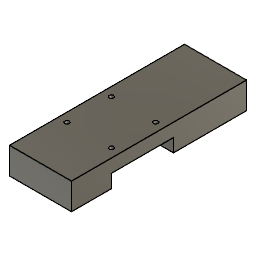
assembly (Autodesk Fusion 360 archive; units mm, degrees)
design "2x4_v2"
part number: 2026-04-10-14-49-08-842
Autodesk Fusion 360 part; units mm, degrees
sketch "Sketch1" plane through (0, 0, 0) normal (0, 0, 1) x (1, 0, 0)
  line L0 (0, 0) -> (88.9, 0)
  line L1 (88.9, 0) -> (88.9, 250.825)
  line L2 (88.9, 250.825) -> (0, 250.825)
  line L3 (0, 250.825) -> (0, 0)
  line L4 (0, 57.15) -> (88.9, 57.15)
  line L5 (0, 146.05) -> (88.9, 146.05)
  dimension "d1" = 88.9
  dimension "d2" = 250.825
  dimension "d3" = 57.15
  dimension "d4" = 88.9
  constraint horizontal L0
  constraint vertical L1
  constraint horizontal L2
  constraint vertical L3
  constraint coincident L0.start L3.end
  constraint coincident L3 L4.start
  constraint coincident L1 L4.end
  constraint perpendicular L1 L4
  constraint coincident L3 L5.start
  constraint coincident L1 L5.end
  constraint perpendicular L1 L5
  measures "d1" distance of L0.start L0.end
  measures "d2" distance of L0.end L1.end
  measures "d3" distance of L0 L4
  measures "d4" distance of L4 L5
extrude "Extrude1" add sketch "Sketch1" along normal blind 38.1
extrude "Extrude2" cut sketch "Sketch1" along normal blind 19.05 contours L1 L3 L4 L5
sketch "Sketch2" plane through (0, 0, 19.05) normal (0, 0, -1) x (1, 0, 0)
  line L0 (88.9, -57.15) -> (0, -57.15)
  line L1 (0, -57.15) -> (0, -146.05)
  line L2 (0, -146.05) -> (88.9, -146.05)
  line L3 (88.9, -146.05) -> (88.9, -57.15)
  line L4 (12.7, -133.35) -> (76.2, -133.35)
  line L5 (76.2, -133.35) -> (76.2, -69.85)
  line L6 (76.2, -69.85) -> (12.7, -69.85)
  line L7 (12.7, -69.85) -> (12.7, -133.35)
  dimension "d9" = -12.7
hole "Hole1" at (76.2, 69.85, 19.05) at (76.2, 133.35, 19.05) at (12.7, 133.35, 19.05) at (12.7, 69.85, 19.05) direction (0, 0, 1) diameter 6.35 depth 25.4 tip angle 118

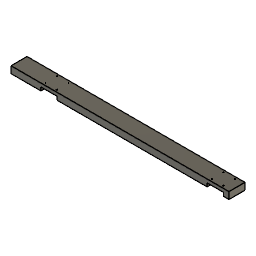
design "2x4_h"
part number: 2026-04-10-14-34-32-967
Autodesk Fusion 360 part; units mm, degrees
sketch "Sketch1" plane through (0, 0, 0) normal (0, 0, 1) x (1, 0, 0)
  line L0 (0, 0) -> (1203.325, 0)
  line L1 (1203.325, 0) -> (1203.325, 88.9)
  line L2 (1203.325, 88.9) -> (0, 88.9)
  line L3 (0, 88.9) -> (0, 0)
  line L4 (165.1, 88.9) -> (165.1, 0)
  line L5 (1171.575, 88.9) -> (1171.575, 0)
  line L6 (1082.675, 88.9) -> (1082.675, 0)
  line L7 (254, 88.9) -> (254, 0)
  dimension "d1" = 88.9
  dimension "d2" = 1203.325
  dimension "d3" = 165.1
  dimension "d4" = 31.75
  dimension "d5" = 88.9
  dimension "d6" = 88.9
  constraint horizontal L0
  constraint vertical L1
  constraint horizontal L2
  constraint vertical L3
  constraint coincident L0.start L3.end
  constraint coincident L2 L4.start
  constraint coincident L0 L4.end
  constraint perpendicular L0 L4
  constraint coincident L2 L5.start
  constraint coincident L0 L5.end
  constraint perpendicular L0 L5
  constraint coincident L2 L6.start
  constraint coincident L0 L6.end
  constraint perpendicular L0 L6
  constraint coincident L2 L7.start
  constraint coincident L0 L7.end
  constraint perpendicular L0 L7
  measures "d1" distance of L0.start L2.end
  measures "d2" distance of L0.start L0.end
  measures "d3" distance of L3 L4
  measures "d4" distance of L1 L5
  measures "d5" distance of L5 L6
  measures "d6" distance of L4 L7
extrude "Extrude1" add sketch "Sketch1" along normal blind 38.1
extrude "Extrude2" cut sketch "Sketch1" along normal blind 19.05 contours L0 L2 L4 L7 | L0 L2 L5 L6
sketch "Sketch2" plane through (0, 0, 19.05) normal (0, 0, -1) x (1, 0, 0)
  line L0 (165.1, 0) -> (165.1, -88.9)
  line L1 (165.1, -88.9) -> (254, -88.9)
  line L2 (254, -88.9) -> (254, 0)
  line L3 (254, 0) -> (165.1, 0)
  line L4 (1082.675, -88.9) -> (1171.575, -88.9)
  line L5 (1171.575, -88.9) -> (1171.575, 0)
  line L6 (1171.575, 0) -> (1082.675, 0)
  line L7 (1082.675, 0) -> (1082.675, -88.9)
  line L8 (177.8, -76.2) -> (241.3, -76.2)
  line L9 (241.3, -76.2) -> (241.3, -12.7)
  line L10 (241.3, -12.7) -> (177.8, -12.7)
  line L11 (177.8, -12.7) -> (177.8, -76.2)
  line L12 (1158.875, -76.2) -> (1158.875, -12.7)
  line L13 (1158.875, -12.7) -> (1095.375, -12.7)
  line L14 (1095.375, -12.7) -> (1095.375, -76.2)
  line L15 (1095.375, -76.2) -> (1158.875, -76.2)
  dimension "d11" = -12.7
  dimension "d12" = -12.7
hole "Hole1" at (177.8, 12.7, 19.05) at (241.3, 12.7, 19.05) at (177.8, 76.2, 19.05) at (241.3, 76.2, 19.05) at (1095.375, 12.7, 19.05) at (1158.875, 12.7, 19.05) at (1095.375, 76.2, 19.05) at (1158.875, 76.2, 19.05) direction (0, 0, 1) diameter 6.35 depth 25.4 tip angle 118

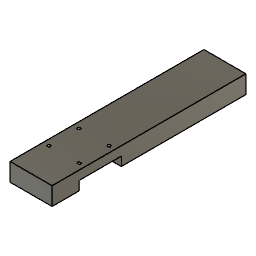
design "2x4_v1"
part number: 2026-04-10-14-49-08-842
Autodesk Fusion 360 part; units mm, degrees
sketch "Sketch1" plane through (0, 0, 0) normal (0, 0, 1) x (1, 0, 0)
  line L0 (0, 0) -> (88.9, 0)
  line L1 (88.9, 0) -> (88.9, 409.575)
  line L2 (88.9, 409.575) -> (0, 409.575)
  line L3 (0, 409.575) -> (0, 0)
  line L4 (0, 57.15) -> (88.9, 57.15)
  line L5 (0, 146.05) -> (88.9, 146.05)
  dimension "d1" = 88.9
  dimension "d2" = 409.575
  dimension "d3" = 57.15
  dimension "d4" = 88.9
  constraint horizontal L0
  constraint vertical L1
  constraint horizontal L2
  constraint vertical L3
  constraint coincident L0.start L3.end
  constraint coincident L3 L4.start
  constraint coincident L1 L4.end
  constraint perpendicular L1 L4
  constraint coincident L3 L5.start
  constraint coincident L1 L5.end
  constraint perpendicular L1 L5
  measures "d1" distance of L0.start L0.end
  measures "d2" distance of L0.end L1.end
  measures "d3" distance of L0 L4
  measures "d4" distance of L4 L5
extrude "Extrude1" add sketch "Sketch1" along normal blind 38.1
extrude "Extrude2" cut sketch "Sketch1" along normal blind 19.05 contours L1 L3 L4 L5
sketch "Sketch2" plane through (0, 0, 19.05) normal (0, 0, -1) x (1, 0, 0)
  line L0 (88.9, -57.15) -> (0, -57.15)
  line L1 (0, -57.15) -> (0, -146.05)
  line L2 (0, -146.05) -> (88.9, -146.05)
  line L3 (88.9, -146.05) -> (88.9, -57.15)
  line L4 (76.2, -69.85) -> (12.7, -69.85)
  line L5 (12.7, -69.85) -> (12.7, -133.35)
  line L6 (12.7, -133.35) -> (76.2, -133.35)
  line L7 (76.2, -133.35) -> (76.2, -69.85)
  dimension "d9" = -12.7
hole "Hole1" at (76.2, 133.35, 19.05) at (12.7, 133.35, 19.05) at (12.7, 69.85, 19.05) at (76.2, 69.85, 19.05) direction (0, 0, 1) diameter 6.35 depth 25.4 tip angle 118
